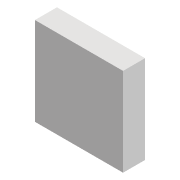
# Autodesk Inventor part: MATERIAL MOLDE 2
Saved by Autodesk Inventor 2021.4 (Build 254397000, 397)
## iProperties
Created: 2023-02-13
Part Number: MATERIAL MOLDE 2
Material: Generic
Document SubType Name: Modeling
Designer: rodar
Density: 1 g/cm^3
Appearance: Default
Author: rodar
Autodesk Inventor part; units mm, degrees
ref_plane "YZ Plane" through (0, 0, 0) normal (1, 0, 0) x (0, 1, 0)
ref_plane "XZ Plane" through (0, 0, 0) normal (0, 1, 0) x (-1, 0, 0)
sketch "Sketch1" plane through (0, 0, 0) normal (0, 0, 1) x (1, 0, 0)
  line L0 (0, 76.2) -> (0, 0) projected
  line L1 (76.2, 76.2) -> (0, 76.2) projected
  line L2 (76.2, 0) -> (76.2, 76.2) projected
  line L3 (0, 0) -> (76.2, 0) projected
ref_plane "Work Plane1" through (-8.001, -8.001, -19.05) normal (0, 0, 1) x (1, 0, 0)
extrude "Extrusion1" add sketch "Sketch1" against normal up to surface (19.05 mm away)
body "Solid1"
